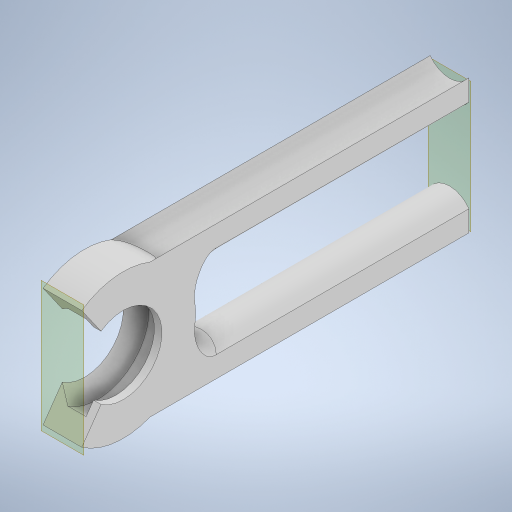
# Autodesk Inventor part: collimator mount
Saved by Autodesk Inventor 2024 (Build 280153000, 153)
## iProperties
Created: 2024-11-08
Part Number: collimator mount
Material: Generic
Document SubType Name: Modeling
Designer: Williamow
Density: 1 g/cm^3
Appearance: Default
Author: Williamow
Autodesk Inventor part; units mm, degrees
ref_plane "YZ Plane" through (0, 0, 0) normal (1, 0, 0) x (0, 1, 0)
ref_plane "XZ Plane" through (0, 0, 0) normal (0, 1, 0) x (-1, 0, 0)
ref_plane "XY Plane" through (0, 0, 0) normal (0, 0, 1) x (1, 0, 0)
sketch "Sketch3" plane through (0, 0, 0) normal (0, 1, 0) x (-1, 0, 0)
  line L0 (0, 0) -> (1.832, 0)
  line L1 (1.5, -1.5) -> (1, -2)
  line L2 (1, -2) -> (0.29, -2)
  line L3 (0.29, -2) -> (0.29, -1.5)
  line L4 (0.29, -1.5) -> (0, -1.5)
  line L5 (0, -1.5) -> (0, -2.8)
  line L6 (0, -2.8) -> (1.5, -2.8)
  line L7 (1.5, -2.8) -> (1.5, -1.5)
  dimension "d10" = 0.5
  dimension "d11" = 45
  dimension "d12" = 0.8
  dimension "d13" = 0.71
  dimension "d14" = 2
  dimension "d22" = 1.5
  constraints: 16 end point, 5 perpendicular, 2 horizontal, 1 horizontal alignment, 1 vertical alignment
  measures "d10" distance of L2.end L3.end
  measures "d11" angle of L7 L1
  measures "d12" distance from line of L6 L2.end
  measures "d13" distance of L1.end L2.end
  measures "d14" distance from line of L0 L2.end
  measures "d22" distance of L5.end L6.end
revolve "Revolution1" add sketch "Sketch3" angle 250 mid plane about axis through (0, 0, 0) along (-1, 0, 0)
ref_plane "Work Plane2" through (0, -2.2936, -13.394) normal (0, 0, -1) x (-1, 0, 0)
ref_plane "Work Plane1" through (0, -2.2936, 1.606) normal (0, 0, -1) x (-1, 0, 0)
sketch "Sketch5" plane through (0, -2.2936, -13.394) normal (0, 0, -1) x (-1, 0, 0)
  line L0 (0, -0.5064) -> (0, 5.0936) projected
  line L1 (1.5, -0.5064) -> (1.5, 5.0936) projected
  arc A0 (0, 4.0836) -> (1.5, 4.0836) centre (0.75, 4.6098) ccw
  arc A1 (0, 4.8936) -> (1.5, 4.8936) centre (0.75, 5.4198) ccw
  line L2 (0, 2.2936) -> (1.5, 2.2936)
  arc A2 (1.5, 0.5036) -> (0, 0.5036) centre (0.75, -0.0225) ccw
  arc A3 (1.5, -0.3064) -> (0, -0.3064) centre (0.75, -0.8325) ccw
  line L3 (0, 4.8936) -> (0.75, 4.8936) construction
  line L4 (0.75, 4.8936) -> (0.75, 3.6936) construction
  point P0 (0, 4.5873)
  point P1 (0, 0)
  point P2 (1.5, 4.5873)
  point P3 (1.5, 0)
  point P4 (0.75, 2.2936)
  point P5 (0.75, 4.2936)
  point P6 (0, -0.3064)
  point P7 (1.5, -0.3064)
  point P8 (1.5, 0.5036)
  point P9 (0, 0.5036)
  point P10 (0.75, 4.2936)
  dimension "d38" = 0.81
  dimension "d45" = 2
  dimension "d46" = 1.2
  constraints: 9 point on circle, 6 end point, 6 symmetric about line, 4 centre point, 4 point on line, 3 midpoint, 2 horizontal alignment, 1 equal radius, 1 horizontal, 1 vertical, 2 other
  measures "d38" distance of L3.start A0.start
  measures "d45" distance of point (0.75, 2.294) point (0.75, 4.294)
  measures "d46" distance of L3.end L4.end
extrude "Extrusion5" add sketch "Sketch5" against normal up to next contours L0 A2 L1 A3 | L0 A1 L1 A0
fillet "Fillet3" radius 1 2 edges at (-0.7504, -1.4, -2.4249) (-0.7496, 1.4, -2.4249)
sketch "Sketch4" plane through (-1.5, 0, 0) normal (-1, 0, 0) x (0, 0, 1)
  arc A0 (1.606, 2.2936) -> (1.606, -2.2936) centre (0, 0) ccw projected
  line L0 (-11.437, 2.4031) -> (-11.437, 1.5969)
  line L1 (-2.3, 1.5969) -> (-3.437, 1.5969)
  line L2 (-3.437, 1.5969) -> (-4.437, 1.4719)
  line L3 (-4.437, 1.4719) -> (-9.437, 1.4719)
  line L4 (-9.437, 1.4719) -> (-10.437, 1.5969)
  line L5 (-10.437, 1.5969) -> (-11.437, 1.5969)
  line L6 (-11.437, 2.4031) -> (-10.437, 2.4031)
  line L7 (-10.437, 2.4031) -> (-9.437, 2.5281)
  line L8 (-9.437, 2.5281) -> (-4.437, 2.5281)
  line L9 (-4.437, 2.5281) -> (-3.437, 2.4031)
  line L10 (-3.437, 2.4031) -> (-1.437, 2.4031)
  line L11 (-3.437, 2) -> (-4.437, 2.125)
  line L12 (-4.437, 2.125) -> (-9.437, 2.125)
  line L13 (-9.437, 2.125) -> (-10.437, 2)
  line L14 (-10.437, 2) -> (-9.437, 1.875)
  line L15 (-9.437, 1.875) -> (-4.437, 1.875)
  line L16 (-4.437, 1.875) -> (-3.437, 2)
  line L17 (0, 0) -> (1.8598, 0)
  line L18 (-11.437, -2.4031) -> (-11.437, -1.5969)
  line L19 (-2.3, -1.5969) -> (-3.437, -1.5969)
  line L20 (-3.437, -1.5969) -> (-4.437, -1.4719)
  line L21 (-4.437, -1.4719) -> (-9.437, -1.4719)
  line L22 (-9.437, -1.4719) -> (-10.437, -1.5969)
  line L23 (-10.437, -1.5969) -> (-11.437, -1.5969)
  line L24 (-11.437, -2.4031) -> (-10.437, -2.4031)
  line L25 (-10.437, -2.4031) -> (-9.437, -2.5281)
  line L26 (-9.437, -2.5281) -> (-4.437, -2.5281)
  line L27 (-4.437, -2.5281) -> (-3.437, -2.4031)
  line L28 (-3.437, -2.4031) -> (-1.437, -2.4031)
  line L29 (-3.437, -2) -> (-4.437, -2.125)
  line L30 (-4.437, -2.125) -> (-9.437, -2.125)
  line L31 (-9.437, -2.125) -> (-10.437, -2)
  line L32 (-10.437, -2) -> (-9.437, -1.875)
  line L33 (-9.437, -1.875) -> (-4.437, -1.875)
  line L34 (-4.437, -1.875) -> (-3.437, -2)
  point P0 (0, 0)
  point P1 (-2.2978, -1.6)
  point P2 (-1.3043, -2.4777)
  point P3 (-11.437, 2)
  point P4 (-11.437, -2)
  point P5 (-1.437, -2.4031)
  dimension "d19" = 10
  dimension "d24" = 1
  dimension "d25" = 2
  dimension "d27" = 1
  dimension "d30" = 2
  dimension "d34" = 0.25
  dimension "d35" = 0.4
  dimension "d36" = 0.4
  constraints: 70 end point, 19 symmetric about line, 7 vertical alignment, 6 parallel, 5 equal length, 4 horizontal, 4 point on circle, 4 point on line, 2 collinear, 1 midpoint, 1 vertical
  measures "d19" distance of L10.end L0.start
  measures "d24" distance of L0.start L6.end
  measures "d25" distance of L9.end L10.end
  measures "d27" horizontal distance of L7.end L6.end
  measures "d30" vertical distance of point (0, 0) point (-11.437, 2)
  measures "d34" distance between parallel lines of L12 L15
  measures "d35" distance between parallel lines of L7 L13
  measures "d36" distance between parallel lines of L4 L14
sketch "Sketch1" plane through (0, 0, 0) normal (0, 1, 0) x (-1, 0, 0)
  line L0 (-0.75, 1.5) -> (0, 2.25)
  line L1 (0, 2.25) -> (0.75, 1.5)
  line L2 (0.75, 1.5) -> (0.95, 1.5)
  line L3 (0.95, 1.5) -> (0.95, 3.5)
  line L4 (0.95, 3.5) -> (-0.95, 3.5)
  line L5 (-0.95, 3.5) -> (-0.95, 1.5)
  line L6 (-0.95, 1.5) -> (-0.75, 1.5)
  line L7 (0, 0) -> (1.8985, 0)
  line L8 (-0.75, -1.5) -> (0, -2.25)
  line L9 (0, -2.25) -> (0.75, -1.5)
  line L10 (0.75, -1.5) -> (0.95, -1.5)
  line L11 (0.95, -1.5) -> (0.95, -3.5)
  line L12 (0.95, -3.5) -> (-0.95, -3.5)
  line L13 (-0.95, -3.5) -> (-0.95, -1.5)
  line L14 (-0.95, -1.5) -> (-0.75, -1.5)
  dimension "d0" = 2.25
  dimension "d1" = 0.2
  dimension "d2" = 2
  dimension "d3" = 1.5
  constraints: 30 end point, 7 symmetric about line, 5 perpendicular, 2 equal length, 2 horizontal, 2 point on line, 1 horizontal alignment, 1 vertical alignment
  measures "d0" distance of L7.start L0.end
  measures "d1" distance of L1.end L2.end
  measures "d2" distance of L2.end L3.end
  measures "d3" distance of L0.start L1.end
sketch "Sketch2" plane through (-0.95, 0, 3.5) normal (0, 0, 1) x (1, 0, 0)
  line L0 (0, 7) -> (1.9, 7) projected
  line L1 (0, 0) -> (0, 7) projected
  line L2 (0, 7) -> (0, 8.5)
  line L3 (0, 8.5) -> (4.4981, 8.5)
  line L4 (4.4981, 8.5) -> (1.9, 7)
  point P0 (0.95, 0)
  dimension "d6" = 30
  dimension "d7" = 1.5
  constraints: 6 end point, 1 perpendicular, 1 vertical
  measures "d6" angle of L4 L3
  measures "d7" distance of L0.start L2.end
body "Solid1"
body "Solid2"
